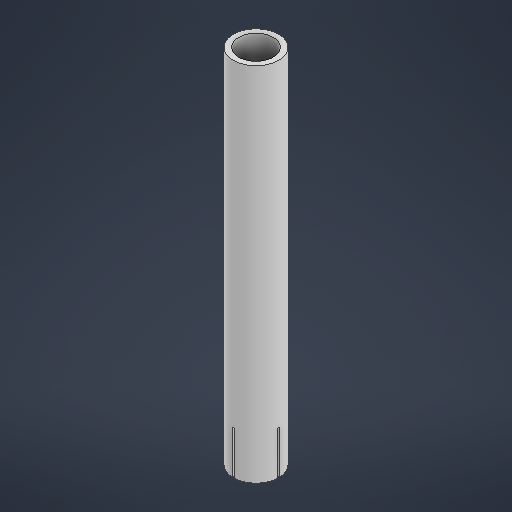
# Autodesk Inventor part: Turret_extend
Saved by Autodesk Inventor 2026.2 (Build 302298010, 298A)
## iProperties
Created: 2026-07-24
Part Number: Turret_extend
Material: Generic
Document SubType Name: Modeling
Designer: vicke
Density: 1 g/cm^3
Appearance: Default
Author: vicke
Autodesk Inventor part; units mm, degrees
ref_plane "YZ Plane" through (0, 0, 0) normal (1, 0, 0) x (0, 1, 0)
ref_plane "XZ Plane" through (0, 0, 0) normal (0, 1, 0) x (-1, 0, 0)
ref_plane "XY Plane" through (0, 0, 0) normal (0, 0, 1) x (1, 0, 0)
sketch "Sketch1" plane through (0, 0, 0) normal (0, 1, 0) x (-1, 0, 0)
  circle A0 centre (0, 0) radius 4.75
  circle A1 centre (0, 0) radius 6.25
  dimension "d0" = 9.5
  dimension "d1" = 1.5
  constraints: 2 centre point, 2 coincident
  measures "d0" diameter of A0
  measures "d1" radial gap between concentric circles of A1 A0
extrude "Extrusion1" add sketch "Sketch1" along normal blind 100
sketch "Sketch2" plane through (0, 0, 0) normal (0, -1, 0) x (1, 0, 0)
  line L0 (-6.25, -0.2) -> (6.25, -0.2)
  line L1 (6.25, -0.2) -> (6.25, 0.2)
  line L2 (6.25, 0.2) -> (-6.25, 0.2)
  line L3 (-6.25, 0.2) -> (-6.25, -0.2)
  line L4 (-0.2, 6.25) -> (-0.2, -6.25)
  line L5 (0.2, -6.25) -> (0.2, 6.25)
  line L6 (-0.2, -6.25) -> (0.2, -6.25)
  line L7 (0.2, 6.25) -> (-0.2, 6.25)
  line L8 (-6.25, -0.2) -> (6.25, -0.2)
  line L9 (6.25, 0.2) -> (-6.25, 0.2)
  line L10 (6.25, -0.2) -> (6.25, 0.2)
  line L11 (-6.25, 0.2) -> (-6.25, -0.2)
  line L12 (0.2, -6.25) -> (0.2, 6.25)
  line L13 (-0.2, 6.25) -> (-0.2, -6.25)
  line L14 (0.2, 6.25) -> (-0.2, 6.25)
  line L15 (-0.2, -6.25) -> (0.2, -6.25)
  point P0 (0, 0)
  point P1 (0.2, -0.2)
  point P2 (0.2, 0.2)
  point P3 (-0.2, 0.2)
  point P4 (-0.2, -0.2)
  dimension "d4" = 12.5
  dimension "d5" = 6.25
  dimension "d6" = 0.4
  dimension "d7" = 0.2
  dimension "d10" = 360
  constraints: 32 end point, 2 parallel, 1 horizontal, 1 perpendicular, 33 other
  measures "d4" distance between parallel lines of L1 L3
  measures "d5" distance from line of point (0, 0) L3
  measures "d6" distance between parallel lines of L2 L0
  measures "d7" distance from line of L2 point (0, 0)
extrude "Extrusion2" cut sketch "Sketch2" against normal blind 12
fillet "Fillet1" radius 1.2 4 edges at (-3.3588, 0, -3.3588) (3.3588, 0, -3.3588) (3.3588, 0, 3.3588) (-3.3588, 0, 3.3588)
body "Solid1"
